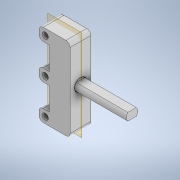
# Autodesk Inventor part: STUURAS
Saved by Autodesk Inventor 2022 (Build 260153000, 153)
## iProperties
Created: 2021-12-21
Part Number: STUURAS
Material: Generic
Document SubType Name: Modeling
Designer: keemi
Density: 1 g/cm^3
Appearance: Default
Author: keemi
Autodesk Inventor part; units mm, degrees
ref_plane "YZ Plane" through (0, 0, 0) normal (1, 0, 0) x (0, 1, 0)
ref_plane "XZ Plane" through (0, 0, 0) normal (0, 1, 0) x (-1, 0, 0)
sketch "Sketch1" plane through (0, 0, 0) normal (0, 1, 0) x (-1, 0, 0)
  line L0 (0, 0) -> (10, 0)
  line L1 (10, 0) -> (10, -10)
  line L2 (10, -10) -> (0, -10)
  line L3 (0, -10) -> (0, 0)
  dimension "d0" = 10
  dimension "d1" = 10
  constraints: 8 end point, 2 parallel, 1 horizontal, 1 perpendicular
  measures "d0" distance of L1.end L2.end
  measures "d1" distance of L0.end L1.end
extrude "Extrusion1" add sketch "Sketch1" along normal blind 40
sketch "Sketch2" plane through (-10, 0, -10) normal (-1, 0, 0) x (0, 0, 1)
  line L0 (0, 40) -> (10, 40) projected
  line L1 (10, 40) -> (0, 40)
  line L2 (0, 40) -> (0, 34)
  line L3 (0, 34) -> (10, 34)
  line L4 (10, 34) -> (10, 40)
  point P0 (10, 0)
  dimension "d4" = 10
  dimension "d5" = 6
  constraints: 8 end point, 2 parallel, 1 horizontal, 1 perpendicular
  measures "d4" distance of L3.end L2.end
  measures "d5" distance of L2.end L1.end
extrude "Extrusion2" add sketch "Sketch2" along normal blind 5
sketch "Sketch3" plane through (-10, 0, -10) normal (-1, 0, 0) x (0, 0, 1)
  line L0 (10, 0) -> (10, 40) projected
  line L1 (10, 0) -> (0, 0)
  line L2 (0, 0) -> (0, 6)
  line L3 (0, 6) -> (10, 6)
  line L4 (10, 6) -> (10, 0)
  dimension "d8" = 10
  dimension "d9" = 6
  constraints: 8 end point, 2 parallel, 1 horizontal, 1 perpendicular
  measures "d8" distance of L2.end L3.end
  measures "d9" distance of L1.end L2.end
extrude "Extrusion3" add sketch "Sketch3" along normal blind 5
sketch "Sketch4" plane through (-10, 34, -10) normal (-1, 0, 0) x (0, 0, 1)
  line L0 (10, -34) -> (10, 6) projected
  line L1 (10, -34) -> (10, -14)
  line L2 (10, -14) -> (10, -17)
  line L3 (10, -17) -> (0, -17)
  line L4 (0, -17) -> (0, -11)
  line L5 (0, -11) -> (10, -11)
  line L6 (10, -11) -> (10, -17)
  point P0 (10, -11)
  dimension "d12" = 20
  dimension "d13" = 3
  dimension "d14" = 10
  dimension "d15" = 6
  constraints: 12 end point, 2 parallel, 1 horizontal, 1 midpoint, 1 perpendicular, 1 point on line
  measures "d12" distance of L0.start L1.end
  measures "d13" distance of L1.end L2.end
  measures "d14" distance of L4.end L5.end
  measures "d15" distance of L3.end L4.end
extrude "Extrusion4" add sketch "Sketch4" along normal blind 5
sketch "Sketch5" plane through (0, 0, 0) normal (0, 0, 1) x (1, 0, 0)
  line L0 (-15, 0) -> (-15, 6) projected
  line L1 (-15, 3) -> (-12, 3)
  line L2 (-15, 23) -> (-15, 17) projected
  line L3 (-15, 20) -> (-12, 20)
  line L4 (-15, 34) -> (-15, 40) projected
  line L5 (-15, 37) -> (-12, 37)
  point P0 (0, 0)
  dimension "d18" = 3
  dimension "d19" = 3
  dimension "d20" = 3
  constraints: 6 end point, 3 horizontal, 3 midpoint
  measures "d18" distance of L1.start L1.end
  measures "d19" distance of L3.start L3.end
  measures "d20" distance of L5.start L5.end
hole "Hole1" at (-12, 37, 0) at (-12, 20, 0) at (-12, 3, 0) direction (0, 0, -1) diameter 3 end through all
fillet "Fillet1" radius 2 8 edges at (-15, 17, -5) (-15, 23, -5) (-15, 40, -5) (-15, 34, -5) (-15, 6, -5) (-15, 0, -5) (0, 40, -5) (0, 0, -5)
sketch "Sketch6" plane through (0, 2, -10) normal (1, 0, 0) x (0, 0, -1)
  point P0 (-10, -2)
sketch "Sketch7" plane through (0, 0, 0) normal (0, 0, 1) x (1, 0, 0)
  point P0 (0, 0)
ref_plane "Work Plane1" through (0, 0, -5) normal (0, 0, 1) x (1, 0, 0)
sketch "Sketch8" plane through (0, 0, -5) normal (0, 0, 1) x (1, 0, 0)
  arc A0 (0, 38) -> (-2, 40) centre (-2, 38) ccw projected
  arc A1 (-2, 0) -> (0, 2) centre (-2, 2) ccw projected
  line L0 (0, 38) -> (0, 2)
  line L1 (0, 2) -> (0, 20)
  line L2 (0, 2) -> (0, 38) projected
  line L3 (0, 20) -> (-9, 20)
  line L4 (-9, 20) -> (-9, 23.5)
  line L5 (0, 20) -> (0, 23)
  line L6 (0, 23) -> (-9, 23.5)
  point P0 (0, 0)
  dimension "d30" = 18
  dimension "d31" = 9
  dimension "d32" = 3.5
  dimension "d33" = 3
  constraints: 12 end point, 2 perpendicular, 1 midpoint, 1 point on line, 1 tangent, 1 vertical
  measures "d30" distance of L0.end L1.end
  measures "d31" distance of L1.end L3.end
  measures "d32" distance of L3.end L4.end
  measures "d33" distance of L1.end L5.end
revolve "Revolution1" cut sketch "Sketch8" angle 360 about axis through (0, 20, -5) along (-1, 0, 0)
sketch "Sketch9" plane through (0, 0, -5) normal (0, 0, 1) x (1, 0, 0)
  line L0 (0, 0) -> (0, 20)
  line L1 (0, 2) -> (0, 38) projected
  line L2 (-9, 16.5) -> (-9, 23.5) projected
  line L3 (0, 20) -> (0, 22.75)
  line L4 (0, 23) -> (0, 17) projected
  line L5 (0, 20) -> (-8.75, 20)
  line L6 (-8.75, 20) -> (-8.75, 23.2)
  line L7 (-8.75, 23.2) -> (0, 22.75)
  dimension "d35" = 20
  dimension "d36" = 2.75
  dimension "d37" = 8.75
  dimension "d38" = 3.2
  dimension "d39" = 90
  constraints: 10 end point, 2 perpendicular, 1 midpoint, 1 point on line
  measures "d35" distance of L0.start L0.end
  measures "d36" distance of L0.end L3.end
  measures "d37" distance of L0.end L5.end
  measures "d38" distance of L5.end L6.end
  measures "d39" angle of L5 L6
revolve "Revolution2" add sketch "Sketch9" angle 360 about axis through (0, 20, -5) along (-1, 0, 0)
sketch "Sketch10" plane through (0, 0, -5) normal (0, 0, 1) x (1, 0, 0)
  point P0 (0, 0)
sketch "Sketch11" plane through (0, 20, -5) normal (1, 0, 0) x (0, 0, -1)
  circle A0 centre (0, 0) radius 2.75
  circle A1 centre (0, 0) radius 2.75 projected
  line L0 (2.75, 0) -> (2.75, 1.85)
  line L1 (2.75, 1.85) -> (-3.3615, 1.85)
  line L2 (-3.3615, 1.85) -> (-3.3615, -1.85)
  line L3 (-3.3615, -1.85) -> (2.75, -1.85)
  line L4 (2.75, -1.85) -> (2.75, 1.85)
  point P0 (-5, -20)
  point P1 (-2.0347, -1.85)
  point P2 (2.0347, -1.85)
  point P3 (2.0347, 1.85)
  point P4 (-2.0347, 1.85)
  dimension "d41" = 1.85
  dimension "d42" = 3.7
  constraints: 10 end point, 2 parallel, 2 vertical, 1 centre point, 1 horizontal, 1 horizontal alignment, 1 perpendicular, 1 tangent, 1 other
  measures "d41" distance of L0.start L0.end
  measures "d42" distance of L2.end L1.end
extrude "Extrusion5" add sketch "Sketch11" along normal blind 25 contours A0 L3 L1
body "Solid1"
